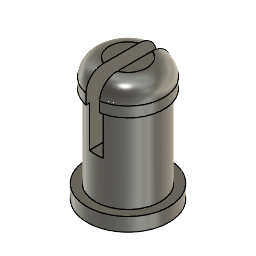
Clip (Autodesk Fusion 360 design; units mm, degrees)
part number: 2026-06-24-10-29-48-035
Autodesk Fusion 360 part; units mm, degrees
note: some values were not read from the file. Set by a fixed rule: which sketch regions a step uses.
sketch "Boceto1" plane through (0, 0, 0) normal (0, 0, 1) x (1, 0, 0)
  circle A0 centre (0, 0) radius 6
  dimension "d1" = 12
  constraint coincident A0.centre origin
  measures "d1" diameter of A0
extrude "Extruir1" add sketch "Boceto1" along normal blind 18
ref_plane "PlanoDeObra1" through (0, 0, 2) normal (0, 0, -1) x (-1, 0, 0)
sketch "Boceto2" plane through (0, 0, 2) normal (0, 0, -1) x (-1, 0, 0)
  circle A0 centre (0, 0) radius 4.75
  circle A1 centre (0, 0) radius 6
  dimension "d5" = 9.5
  dimension "d6" = 12
  constraint coincident A0.centre A1.centre
  measures "d5" diameter of A0
  measures "d6" diameter of A1
extrude "Extruir2" cut sketch "Boceto2" against normal blind 12
sketch "Boceto3" plane through (0, 0, 18) normal (0, 0, 1) x (-1, 0, 0)
  line L0 (-1, 7) -> (1, 7)
  line L1 (1, 7) -> (1, -7)
  line L2 (1, -7) -> (-1, -7)
  line L3 (-1, -7) -> (-1, 7)
  circle A0 centre (0, 0) radius 10
  circle A1 centre (0, 0) radius 6
  circle A2 centre (0, 0) radius 5.25
  circle A3 centre (0, 0) radius 6
  dimension "d11" = 2
  dimension "d12" = 1
  dimension "d15" = 10.5
  dimension "d16" = 12
  constraint horizontal L0
  constraint vertical L1
  constraint horizontal L2
  constraint vertical L3
  constraint coincident A0.centre A1.centre
  constraint concentric A0 A2
  constraint concentric A2 A3
  measures "d11" distance of L1.end L2.end
  measures "d12" distance of A0.centre L1
  measures "d15" diameter of A2
  measures "d16" diameter of A3
extrude "Extruir3" cut sketch "Boceto3" against normal blind 10 contours L0 L1 L3 A1 A3 | L1 L3 A1 A2 A3 | L3 A1 A2 A3 | L1 A1 A2 A3 | L1 L3 A2 | L1 L2 L3 A1 A3 | L1 L3 A1 A2 A3
fillet "Empalme3" radius 2.5 2 edges at (5.25, 0, 18) (-5.25, 0, 18)
